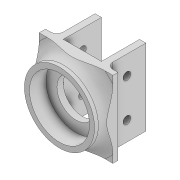
# Autodesk Inventor part: Bearing holder
Saved by Autodesk Inventor 2022 (Build 260153000, 153)
## iProperties
Created: 2024-04-01
Part Number: Bearing holder
Material: Generic
Document SubType Name: Modeling
Designer: LaptopJR
Density: 1 g/cm^3
Appearance: Default
Author: LaptopJR
## iProperties of the stored document Bearing holder_3DPrint.ipt
Created: 2024-04-08
Part Number: Bearing holder_3DPrint
Material: Generic
Document SubType Name: Modeling
Designer: LaptopJR
Density: 1 g/cm^3
Appearance: Default
Author: LaptopJR
Autodesk Inventor part; units mm, degrees
ref_plane "YZ Plane" through (0, 0, 0) normal (1, 0, 0) x (0, 1, 0)
ref_plane "XZ Plane" through (0, 0, 0) normal (0, 1, 0) x (-1, 0, 0)
ref_plane "XY Plane" through (0, 0, 0) normal (0, 0, 1) x (1, 0, 0)
sketch "Sketch1" plane through (0, 0, 0) normal (0, 1, 0) x (-1, 0, 0)
  line L0 (0, 0) -> (-30, 0)
  line L1 (-30, 0) -> (-30, -30)
  line L2 (-30, -30) -> (0, -30)
  line L3 (0, -30) -> (0, 0)
  line L4 (-35, -35) -> (-35, 5)
  line L5 (-35, 5) -> (5, 5)
  line L6 (5, 5) -> (5, -35)
  line L7 (5, -35) -> (-35, -35)
  line L8 (0, -30) -> (5, -30)
  line L9 (-30, -30) -> (-35, -30)
  dimension "d0" = 30
  dimension "d1" = 30
  dimension "d2" = 5
  constraints: 20 end point, 4 parallel, 3 horizontal, 2 perpendicular, 2 point on line, 3 other
  measures "d0" distance of L2.end L1.end
  measures "d1" distance of L1.end L0.end
  measures "d2" distance between parallel lines of L1 L4
extrude "Extrusion1" add sketch "Sketch1" along normal blind 60 contours L0 L1 L9 L4 L5 L6 L8 L3
sketch "Sketch2" plane through (-5, 0, 5) normal (0, 0, 1) x (1, 0, 0)
  line L0 (0, 0) -> (40, 0) projected
  line L1 (40, 0) -> (40, 60) projected
  line L2 (0, 60) -> (40, 60) projected
  line L3 (0, 0) -> (0, 60) projected
  line L4 (0, 60) -> (40, 60) projected
  line L5 (0, 0) -> (40, 0) projected
  line L6 (0, 60) -> (40, 0) construction
  circle A0 centre (20, 30) radius 23.6
  circle A1 centre (20, 30) radius 27.6
  dimension "d5" = 47.2
  dimension "d6" = 4
  constraints: 2 centre point, 2 end point, 1 midpoint
  measures "d5" diameter of A0
  measures "d6" radial gap between concentric circles of A0 A1
extrude "Extrusion2" add sketch "Sketch2" along normal blind 13 contours A1 L3 A0 | L3 A0 L1 A1 | L1 A0 A1 | A1 L1 A0 L3
sketch "Sketch3" plane through (35, 0, 5) normal (1, 0, 0) x (0, 0, -1)
  line L0 (5, 60) -> (35, 60) projected
  line L1 (35, 60) -> (0, 60) projected
  line L2 (5, 0) -> (35, 0) projected
  line L3 (0, 60) -> (4, 60)
  line L4 (4, 60) -> (4, 0)
  line L5 (4, 0) -> (0, 0)
  line L6 (0, 0) -> (0, 60)
  point P0 (4, 60)
  dimension "d10" = 4
  constraints: 8 end point, 2 parallel, 1 horizontal, 1 perpendicular, 1 point on line
  measures "d10" distance of L4.end L5.end
extrude "Extrusion3" add sketch "Sketch3" along normal blind 9
sketch "Sketch4" plane through (-5, 0, -30) normal (-1, 0, 0) x (0, 0, 1)
  line L0 (0, 60) -> (35, 60) projected
  line L1 (30, 0) -> (0, 0) projected
  line L2 (35, 60) -> (30, 60)
  line L3 (30, 60) -> (30, 0)
  line L4 (30, 0) -> (35, 0)
  line L5 (35, 0) -> (35, 60)
  constraints: 8 end point, 2 parallel, 1 horizontal, 1 perpendicular
extrude "Extrusion4" add sketch "Sketch4" along normal blind 9
sketch "Sketch5" plane through (15, 30, 5) normal (0, 0, 1) x (1, 0, 0)
  circle A0 centre (0, 0) radius 23.6 projected
  circle A1 centre (0, 0) radius 15
  point P0 (-15, -30)
  dimension "d15" = 30
  constraints: 1 centre point, 1 coincident
  measures "d15" diameter of A1
extrude "Extrusion5" cut sketch "Sketch5" against normal blind 9 contours A1
fillet "Fillet1" radius 10 1 edges at (-12.6, 30, 5)
sketch "Sketch7" plane through (35, 0, -30) normal (1, 0, 0) x (0, 0, -1)
  line L0 (-31, 60) -> (-31, 0) projected
  line L1 (-31, 0) -> (0, 0) projected
  line L2 (0, 0) -> (0, 60) projected
  line L3 (-31, 60) -> (0, 60) projected
  line L4 (-30, 0) -> (0, 0) projected
  line L5 (-15, 0) -> (-15, 15) construction
  line L6 (-15, 15) -> (-15, 45) construction
  line L7 (-15, 45) -> (-15, 60) construction
  line L8 (0, 60) -> (-31, 60) projected
  circle A0 centre (-15, 15) radius 3.05
  circle A1 centre (-15, 45) radius 3.05
  dimension "d19" = 30
  dimension "d20" = 6.1
  constraints: 6 end point, 2 centre point, 2 coincident, 2 point on line, 1 collinear, 1 equal radius, 1 midpoint, 1 vertical
  measures "d19" distance of L5.end L6.end
  measures "d20" diameter of A1
extrude "Extrusion6" cut sketch "Sketch7" against normal blind 40 contours A0 | A1
fillet "Fillet2" radius 5 2 edges at (-5, 30, 0) (35, 30, 1)
body "Solid1"
